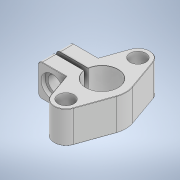
# Autodesk Inventor part: Kep_Truc
Saved by Autodesk Inventor 2022 (Build 260153000, 153)
## iProperties
Created: 2022-11-14
Part Number: Kep_Truc
Material: Generic
Document SubType Name: Modeling
Designer: nguye
Density: 1 g/cm^3
Appearance: Default
Author: nguye
Autodesk Inventor part; units mm, degrees
ref_plane "YZ Plane" through (0, 0, 0) normal (1, 0, 0) x (0, 1, 0)
ref_plane "XZ Plane" through (0, 0, 0) normal (0, 1, 0) x (-1, 0, 0)
ref_plane "XY Plane" through (0, 0, 0) normal (0, 0, 1) x (1, 0, 0)
sketch "Sketch1" plane through (0, 0, 0) normal (0, 1, 0) x (-1, 0, 0)
  circle A0 centre (0, 0) radius 4
  circle A1 centre (0, 0) radius 6
  line L0 (0, 4) -> (12, 4)
  line L1 (12, 4) -> (12, -4)
  line L2 (12, -4) -> (0, -4)
  line L3 (3.9686, 0.5) -> (15, 0.5)
  line L4 (15, 0.5) -> (15, -0.5)
  line L5 (15, -0.5) -> (3.9686, -0.5)
  circle A2 centre (0, 9) radius 2
  circle A3 centre (0, -9) radius 2
  circle A4 centre (0, 9) radius 3
  circle A5 centre (0, -9) radius 3
  line L6 (2.8284, 10) -> (5.6569, 2)
  line L7 (-2.8284, 10) -> (-5.6569, 2)
  line L8 (5.6569, -2) -> (2.8284, -10)
  line L9 (-5.6569, -2) -> (-2.8284, -10)
  point P0 (15, 0)
  point P1 (4.9497, 4)
  point P2 (4.9497, -4)
  point P3 (12, -0.5)
  point P4 (12, 0.5)
  dimension "d0" = 8
  dimension "d1" = 12
  dimension "d2" = 8
  dimension "d3" = 12
  dimension "d4" = 1
  dimension "d5" = 15
  dimension "d6" = 4
  dimension "d7" = 4
  dimension "d8" = 18
  dimension "d9" = 9
  dimension "d10" = 6
  dimension "d11" = 6
  constraints: 20 end point, 12 point on circle, 7 tangent, 6 centre point, 4 coincident, 4 perpendicular, 3 vertical alignment, 2 horizontal, 1 horizontal alignment, 1 midpoint, 1 parallel
  measures "d0" diameter of A0
  measures "d1" diameter of A1
  measures "d2" distance of L0.end L1.end
  measures "d3" distance from line of point (0, 0) L1
  measures "d4" distance between parallel lines of L5 L3
  measures "d5" distance of point (15, 0) point (0, 0)
  measures "d6" diameter of A2
  measures "d7" diameter of A3
  measures "d8" distance of A3.centre A2.centre
  measures "d9" distance of point (0, 0) A3.centre
  measures "d10" diameter of A4
  measures "d11" diameter of A5
extrude "Extrusion1" add sketch "Sketch1" along normal blind 8 contours A0 L0 A1 L3 | L5 A1 L2 A0 | A0 L2 A1 L0 | A1 L6 L0 L1 L3 | L5 L1 L2 L8 A1 | L0 L6 A1 | A1 A4 L6 L0 | L2 L8 A5 A1 | A1 L8 L2 | A1 L7 A4 | A4 | A5 L9 A1 | A5
sketch "Sketch2" plane through (-4.9497, 0, -4) normal (0, 0, -1) x (-1, 0, 0)
  circle A0 centre (3.5503, 4) radius 2
  line L0 (7.0503, 0) -> (7.0503, 8) projected
  circle A1 centre (3.5503, 4) radius 2.75
  line L1 (0, 8) -> (7.0503, 8) projected
  circle A2 centre (6.0503, 7) radius 1
  circle A3 centre (6.0503, 1) radius 1
  line L2 (0, 0) -> (7.0503, 0) projected
  point P0 (-4.9497, 0)
  point P1 (7.0503, 4)
  point P2 (6.0503, 0)
  point P3 (7.0503, 1)
  point P4 (6.0503, 8)
  point P5 (7.0503, 7)
  dimension "d14" = 4
  dimension "d15" = 3.5
  dimension "d18" = 5.5
  dimension "d19" = 2
  dimension "d20" = 2
  constraints: 4 centre point, 4 tangent, 1 coincident, 1 horizontal alignment, 1 midpoint
  measures "d14" diameter of A0
  measures "d15" distance from line of L0 A0.centre
  measures "d18" diameter of A1
  measures "d19" diameter of A2
  measures "d20" diameter of A3
extrude "Extrusion2" cut sketch "Sketch2" against normal blind 8 contours A0 | L2 A3 L0 | A2 L1 L0
sketch "Sketch3" plane through (-4.9497, 0, -4) normal (0, 0, -1) x (-1, 0, 0)
  circle A0 centre (3.5503, 4) radius 2 projected
  circle A1 centre (3.5503, 4) radius 2.75
  point P0 (-4.9497, 0)
  dimension "d21" = 5.5
  constraints: 1 centre point, 1 coincident
  measures "d21" diameter of A1
extrude "Extrusion3" cut sketch "Sketch3" against normal blind 1
mirror "Mirror1" about plane through (0, 0, 0) normal (0, 0, 1) of "Extrusion3"
chamfer "Chamfer1" distance 0.1 angle 45 24 edges at (-7.9749, 8, 4) (-11.7071, 7.7071, 4) (-12, 4, 4) (-11.7071, 0.2929, 4) (-7.9749, 0, 4) (-3.8891, 8, 7) (0, 8, 12) (4.2426, 8, 6) (6, 8, 0) (4.2426, 8, -6) (0, 8, -12) (-3.8891, 8, -7) (-7.9749, 8, -4) (-11.7071, 7.7071, -4) (-12, 4, -4) (-11.7071, 0.2929, -4) (-7.9749, 0, -4) (4.2426, 0, 6) (6, 0, 0) (4.2426, 0, -6) (0, 0, -12) (-3.8891, 0, -7) (0, 0, 12) (-3.8891, 0, 7)
chamfer "Chamfer2" distance 0.05 angle 45 12 edges at (-7.4843, 8, 0.5) (-11.7071, 7.7071, 0.5) (-12, 4, 0.5) (-11.7071, 0.2929, 0.5) (-7.4843, 0, 0.5) (-7.4843, 8, -0.5) (-11.7071, 7.7071, -0.5) (-12, 4, -0.5) (-11.7071, 0.2929, -0.5) (-7.4843, 0, -0.5) (4, 8, 0) (4, 0, 0)
body "Solid1"
